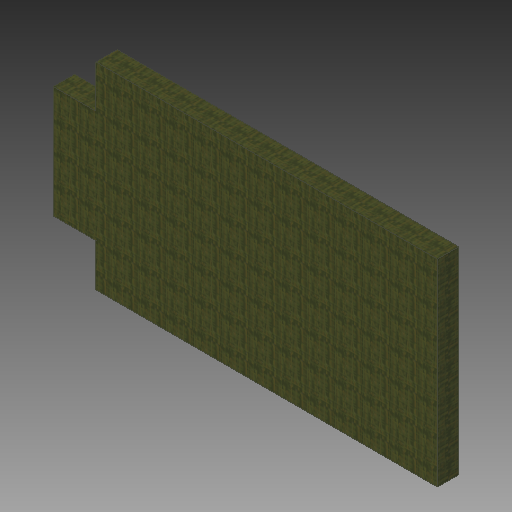
# Autodesk Inventor part: 1214_Gantry Support Rib_V1
Saved by Autodesk Inventor 2020 (Build 240168000, 168)
## iProperties
Created: 2017-08-30
Part Number: 1214_Gantry Support Rib_V1
Material: GFRP
Document SubType Name: Modeling
Designer: e22ma
Density: 1.75 g/cm^3
Appearance: Smooth - Light Gray
Mass: 568.17 g
Surface Area: 599.192 cm^2
Volume: 324.669 cm^3
Author: e22ma
Autodesk Inventor part; units mm, degrees
ref_plane "YZ Plane" through (0, 0, 0) normal (1, 0, 0) x (0, 1, 0)
ref_plane "XZ Plane" through (0, 0, 0) normal (0, 1, 0) x (-1, 0, 0)
ref_plane "XY Plane" through (0, 0, 0) normal (0, 0, 1) x (1, 0, 0)
sketch "Sketch1" plane through (0, 0, 0) normal (0, 0, 1) x (1, 0, 0)
  line L0 (-101.6, -58.7375) -> (101.6, -58.7375)
  line L1 (101.6, -58.7375) -> (101.6, 58.7375)
  line L2 (101.6, 58.7375) -> (-101.6, 58.7375)
  line L3 (-101.6, 58.7375) -> (-101.6, -58.7375)
  line L4 (-101.6, -58.7375) -> (101.6, 58.7375) construction
  line L5 (101.6, -58.7375) -> (-101.6, 58.7375) construction
  line L6 (-101.6, -33.3375) -> (-101.6, 33.3375)
  line L7 (-101.6, 33.3375) -> (-127, 33.3375)
  line L8 (-127, 33.3375) -> (-127, -33.3375)
  line L9 (-127, -33.3375) -> (-101.6, -33.3375)
  point P0 (0, 0)
  dimension "d0" = 203.2
  dimension "d1" = 117.475
  dimension "d2" = 25.4
  dimension "d3" = 25.4
  dimension "d4" = 25.4
  constraints: 20 end point, 4 parallel, 2 midpoint, 2 perpendicular, 2 point on line, 1 horizontal
  measures "d0" distance of L2.end L1.end
  measures "d1" distance of L1.end L0.end
  measures "d2" distance between parallel lines of L0 L9
  measures "d3" distance between parallel lines of L2 L7
  measures "d4" distance between parallel lines of L3 L8
extrude "Extrusion1" add sketch "Sketch1" along normal mid plane 12.7
body "Solid1"
